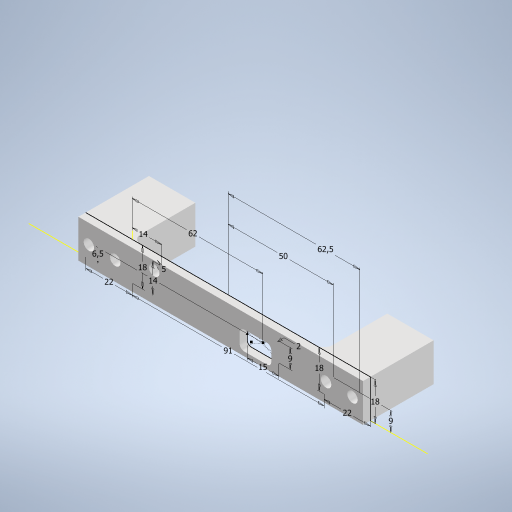
# Autodesk Inventor part: camera_holder
Saved by Autodesk Inventor 2024.3 (Build 283343000, 343)
## iProperties
Created: 2026-05-02
Part Number: camera_holder
Material: Generic
Document SubType Name: Modeling
Designer: owozn
Density: 1 g/cm^3
Appearance: Default
Author: owozn
Autodesk Inventor part; units mm, degrees
ref_plane "YZ Plane" through (0, 0, 0) normal (1, 0, 0) x (0, 1, 0)
ref_plane "XZ Plane" through (0, 0, 0) normal (0, 1, 0) x (-1, 0, 0)
ref_plane "XY Plane" through (0, 0, 0) normal (0, 0, 1) x (1, 0, 0)
sketch "Sketch3" plane through (0, 0, 0) normal (0, 0, 1) x (1, 0, 0)
  line L0 (0, -3.6) -> (0, 21.6) projected
  line L1 (-49, 0) -> (140, 0) projected
  circle A0 centre (14, 14) radius 2.5
  line L2 (56.5, 11) -> (67.5, 11)
  line L3 (69.5, 9) -> (69.5, 4)
  line L4 (67.5, 2) -> (56.5, 2)
  line L5 (54.5, 4) -> (54.5, 9)
  line L6 (54.5, 11) -> (69.5, 2) construction
  line L7 (69.5, 11) -> (54.5, 2) construction
  arc A1 (69.5, 9) -> (67.5, 11) centre (67.5, 9) ccw
  arc A2 (67.5, 2) -> (69.5, 4) centre (67.5, 4) ccw
  arc A3 (54.5, 4) -> (56.5, 2) centre (56.5, 4) ccw
  arc A4 (56.5, 11) -> (54.5, 9) centre (56.5, 9) ccw
  line L8 (0, 18) -> (91, 18)
  line L9 (91, 18) -> (91, 0)
  line L10 (91, 0) -> (0, 0)
  line L11 (0, 0) -> (0, 18)
  line L12 (0, 18) -> (91, 0) construction
  line L13 (91, 18) -> (0, 0) construction
  line L14 (-22, 18) -> (0, 18)
  line L15 (0, 18) -> (0, 0)
  line L16 (0, 0) -> (-22, 0)
  line L17 (-22, 0) -> (-22, 18)
  line L18 (-22, 18) -> (0, 0) construction
  line L19 (0, 18) -> (-22, 0) construction
  line L20 (45.5, 18) -> (45.5, 0) construction
  line L21 (91, 18) -> (113, 18)
  line L22 (113, 18) -> (113, 0)
  line L23 (113, 0) -> (91, 0)
  line L24 (91, 0) -> (91, 18)
  line L25 (91, 18) -> (113, 0) construction
  line L26 (113, 18) -> (91, 0) construction
  point P0 (0, 0)
  point P1 (62, 6.5)
  point P2 (54.5, 6.5)
  point P3 (45.5, 9)
  point P4 (-11, 9)
  point P5 (102, 9)
  point P6 (-22, 0)
  point P7 (113, 0)
  point P8 (95.5, 9)
  point P9 (108, 9)
  point P10 (-4.5, 9)
  point P11 (-17, 9)
  dimension "d26" = 5
  dimension "d29" = 15
  dimension "d30" = 9
  dimension "d31" = 2
  dimension "d34" = 91
  dimension "d35" = 18
  dimension "d36" = 22
  dimension "d37" = 18
  dimension "d38" = 22
  dimension "d39" = 18
  dimension "d41" = 14
  dimension "d42" = 14
  dimension "d56" = 62
  dimension "d57" = 6.5
  dimension "d60" = 50
  dimension "d61" = 62.5
  dimension "d62" = 9
  constraints: 50 end point, 11 midpoint, 8 parallel, 8 point on circle, 8 point on line, 8 tangent, 6 collinear, 5 centre point, 4 horizontal, 4 perpendicular, 3 equal radius, 2 symmetric about line, 1 horizontal alignment
  measures "d26" diameter of A0
  measures "d29" distance of L6.end L7.end
  measures "d30" distance of L7.start L6.end
  measures "d31" radius of A1
  measures "d34" distance of L9.end L10.end
  measures "d35" distance of L8.end L9.end
  measures "d36" distance of L15.end L16.end
  measures "d37" distance of L14.end L15.end
  measures "d38" distance of L22.end L23.end
  measures "d39" distance of L21.end L22.end
  measures "d41" distance from line of L1 A0.centre
  measures "d42" distance from line of L0 A0.centre
  measures "d56" distance from line of L0 point (62, 6.5)
  measures "d57" distance from line of L1 point (62, 6.5)
  measures "d60" distance from line of point (95.5, 9) L20
  measures "d61" distance from line of point (108, 9) L20
  measures "d62" distance from line of L1 point (95.5, 9)
extrude "Extrusion4" add sketch "Sketch3" along normal blind 3.5
extrude "Extrusion5" add sketch "Sketch3" against normal blind 30 contours L1 L17 L14 L0 | L9 L21 L22 L1
hole "Hole1" at (95.5, 9, 0) at (108, 9, 0) at (-4.5, 9, 0) at (-17, 9, 0) direction (0, 0, -1) diameter 5 end through all both
fillet "Fillet1" radius 4 2 edges at (0, 9, 0) (91, 9, 0)
body "Solid2"
